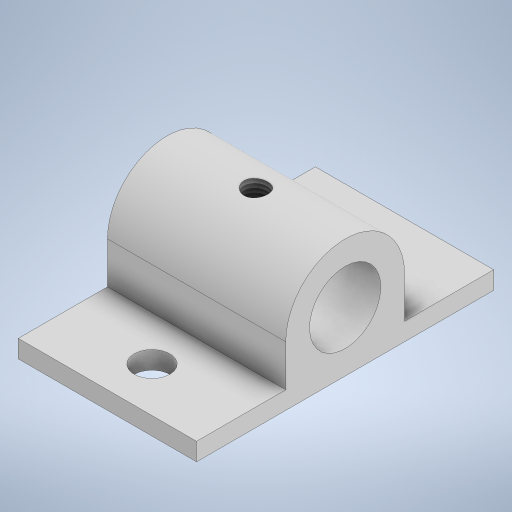
# Autodesk Inventor part: base_axis_static_12mm
Saved by Autodesk Inventor 2024 (Build 280153000, 153)
## iProperties
Created: 2025-12-09
Part Number: base_axis_static_12mm
Material: Generic
Document SubType Name: Modeling
Designer: schar
Density: 1 g/cm^3
Appearance: Default
Author: schar
Autodesk Inventor part; units mm, degrees
ref_plane "YZ Plane" through (0, 0, 0) normal (1, 0, 0) x (0, 1, 0)
ref_plane "XZ Plane" through (0, 0, 0) normal (0, 1, 0) x (-1, 0, 0)
ref_plane "XY Plane" through (0, 0, 0) normal (0, 0, 1) x (1, 0, 0)
sketch "Sketch1" plane through (0, 0, 0) normal (1, 0, 0) x (0, 1, 0)
  circle A0 centre (0, 0) radius 6
  circle A1 centre (0, 0) radius 10
  line L0 (0, 10) -> (-10, 10)
  line L1 (-10, 10) -> (-10, -10)
  line L2 (-10, -10) -> (0, -10)
  line L3 (-10, -10) -> (-7, -10)
  line L4 (-7, -10) -> (-7, -25)
  line L5 (-7, -25) -> (-10, -25)
  line L6 (-10, -25) -> (-10, -10)
  line L7 (-10, 10) -> (-7, 10)
  line L8 (-7, 10) -> (-7, 25)
  line L9 (-7, 25) -> (-10, 25)
  line L10 (-10, 25) -> (-10, 10)
  dimension "d0" = 12
  dimension "d1" = 20
  dimension "d2" = 3
  dimension "d3" = 15
  dimension "d4" = 3
  dimension "d5" = 15
  constraints: 22 end point, 4 parallel, 3 horizontal, 3 perpendicular, 2 centre point, 2 coincident, 2 point on circle, 1 tangent
  measures "d0" diameter of A0
  measures "d1" diameter of A1
  measures "d2" distance of L4.end L5.end
  measures "d3" distance of L3.end L4.end
  measures "d4" distance of L9.end L8.end
  measures "d5" distance of L8.end L7.end
extrude "Extrusion1" add sketch "Sketch1" along normal blind 30
sketch "Sketch2" plane through (0, -7, 25) normal (0, 1, 0) x (1, 0, 0)
  line L0 (0, 0) -> (30, 0) projected
  line L1 (0, 0) -> (15, 0)
  line L2 (15, 0) -> (15, 7.5)
  line L3 (15, 7.5) -> (0, 7.5)
  line L4 (0, 7.5) -> (0, 0)
  line L5 (30, 0) -> (30, 50) projected
  line L6 (30, 50) -> (15, 50)
  line L7 (15, 50) -> (15, 42.5)
  line L8 (15, 42.5) -> (30, 42.5)
  line L9 (30, 42.5) -> (30, 50)
  circle A0 centre (15, 7.5) radius 3
  circle A1 centre (15, 42.5) radius 3
  point P0 (0, 25)
  dimension "d8" = 15
  dimension "d9" = 7.5
  dimension "d10" = 15
  dimension "d11" = 7.5
  dimension "d12" = 6
  dimension "d13" = 6
  constraints: 16 end point, 4 parallel, 2 centre point, 2 coincident, 2 horizontal, 2 perpendicular
  measures "d8" distance of L3.end L2.end
  measures "d9" distance of L2.end L1.end
  measures "d10" distance of L8.end L7.end
  measures "d11" distance of L7.end L6.end
  measures "d12" diameter of A0
  measures "d13" diameter of A1
ref_plane "Work Plane1" through (0, 10, 0) normal (0, 1, 0) x (1, 0, 0)
sketch "Sketch3" plane through (0, 10, 0) normal (0, 1, 0) x (1, 0, 0)
  line L0 (0, 0) -> (15, 0)
  circle A0 centre (15, 0) radius 2
  dimension "d14" = 15
  dimension "d15" = 4
  constraints: 2 end point, 1 centre point, 1 coincident, 1 horizontal
  measures "d14" distance of L0.start L0.end
  measures "d15" diameter of A0
hole "Hole1" at (15, 10, 0) direction (0, -1, 0) diameter 4 depth 8 tip angle 118
thread "Thread1" size "M4x0.7" class "6H" standard "ANSI Metric M Profile" full length
hole "Hole2" at (15, -7, 17.5) at (15, -7, -17.5) direction (0, -1, 0) diameter 6 end through all
body "Solid1"
